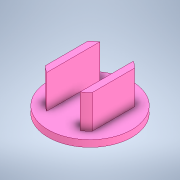
# Autodesk Inventor part: bracketForGarageUpperHalfV02
Saved by Autodesk Inventor 2022.2 (Build 262287000, 287)
## iProperties
Created: 2021-10-20
Part Number: bracketForGarageUpperHalfV02
Material: PC/ABS Plastic
Document SubType Name: Modeling
Designer: robst
Density: 0.357273 g/cm^3
Appearance: Pink
Author: robst
Autodesk Inventor part; units mm, degrees
ref_plane "YZ Plane" through (0, 0, 0) normal (1, 0, 0) x (0, 1, 0)
ref_plane "XZ Plane" through (0, 0, 0) normal (0, 1, 0) x (-1, 0, 0)
ref_plane "XY Plane" through (0, 0, 0) normal (0, 0, 1) x (1, 0, 0)
sketch "Sketch47" plane through (0, 0, 0) normal (0, 1, 0) x (-1, 0, 0)
  circle A0 centre (0, 0) radius 38.1
  dimension "d220" = 76.2
  constraints: 1 centre point, 1 coincident
  measures "d220" diameter of A0
extrude "Extrusion22" add sketch "Sketch47" against normal blind 8
sketch "Sketch48" plane through (0, 0, 0) normal (0, 1, 0) x (1, 0, 0)
  circle A0 centre (0, 0) radius 38.1 projected
  line L0 (-20.32, 32.229) -> (-20.32, -32.229)
  line L1 (20.32, 32.229) -> (20.32, -32.229)
  line L2 (-28.32, 25.487) -> (-28.32, -25.487)
  line L3 (28.32, 25.487) -> (28.32, -25.487)
  arc A1 (-20.32, 32.229) -> (-28.32, 25.487) centre (0, 0) ccw
  arc A2 (-28.32, -25.487) -> (-20.32, -32.229) centre (0, 0) ccw
  arc A3 (20.32, -32.229) -> (28.32, -25.487) centre (0, 0) ccw
  arc A4 (28.32, 25.487) -> (20.32, 32.229) centre (0, 0) ccw
  dimension "d223" = 40.64
  dimension "d224" = 8
  constraints: 8 end point, 8 point on circle, 4 centre point, 4 parallel, 2 vertical, 1 coincident, 9 other
  measures "d223" distance between parallel lines of L1 L0
  measures "d224" distance between parallel lines of L2 L0
extrude "Extrusion23" add sketch "Sketch48" along normal blind 40.64 contours L3 A0 L1 | L0 A0 L2
sketch "Sketch49" plane through (0, -8, 0) normal (0, -1, 0) x (1, 0, 0)
  circle A0 centre (0, 0) radius 38.1 projected
  circle A1 centre (0, 0) radius 38.1
  circle A2 centre (0, 0) radius 50.8
  dimension "d227" = 101.6
  constraints: 2 centre point, 2 coincident, 1 concentric
  measures "d227" diameter of A2
extrude "Extrusion24" add sketch "Sketch49" against normal blind 8
equation "\"d221\" = wallThickness"
equation "\"d223\" = twoByFourWidth"
equation "\"d224\" = wallThickness"
equation "\"d225\" = twoByFourWidth"
equation "\"d228\" = wallThickness"
equation "\"wallThickness\" = 8"
equation "\"twoByFourWidth\" = 40.64"
equation "\"twoByFourDepth\" = 84.1375"
equation "\"azimuth\" = -15deg"
equation "\"elevation\" = 20deg"
equation "\"centerForTwoHoles\" = 0.25 * diagonalLine"
equation "\"depthOfExtrusionForMatingToLowerHalf\" = 12.5"
equation "\"depthForWasherForMatingToCase\" = 14"
equation "\"diagonalLine\" = 85.134222"
body "Solid3"
